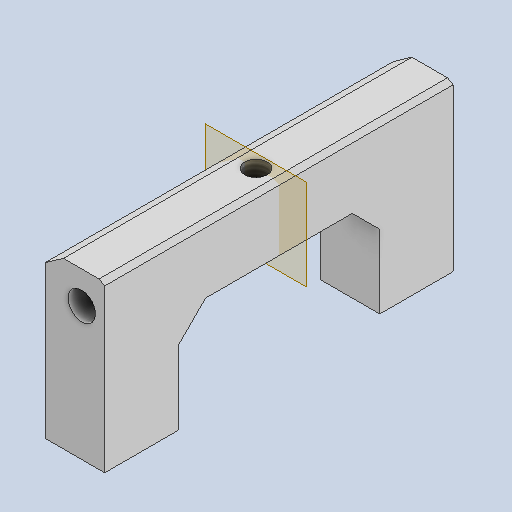
# Autodesk Inventor part: daVincihead_Sled_ToolAufnahmeBuegel_38mm
Saved by Autodesk Inventor 2024 (Build 280153000, 153)
## iProperties
Created: 2022-08-16
Part Number: daVincihead_Sled_ToolAufnahmeBuegel_38mm
Material: Generisch
Document SubType Name: Modeling
Designer: alexw
Density: 1 g/cm^3
Appearance: Vorgabe
Mass: 2.50955 g
Surface Area: 21.9008 cm^2
Volume: 2.50955 cm^3
Author: alexw
Autodesk Inventor part; units mm, degrees
ref_plane "YZ Plane" through (0, 0, 0) normal (1, 0, 0) x (0, 1, 0)
ref_plane "XZ Plane" through (0, 0, 0) normal (0, 1, 0) x (-1, 0, 0)
ref_plane "XY Plane" through (0, 0, 0) normal (0, 0, 1) x (1, 0, 0)
sketch "Skizze1" plane through (0, 0, 0) normal (0, 0, 1) x (1, 0, 0)
  line L0 (-4, 3.5) -> (4, 3.5)
  line L1 (4, 3.5) -> (4, -3.5)
  line L2 (4, -3.5) -> (-4, -3.5)
  line L3 (-4, -3.5) -> (-4, 3.5)
  line L4 (-4, 3.5) -> (4, -3.5) construction
  line L5 (4, 3.5) -> (-4, -3.5) construction
  line L6 (-4, 2.0996) -> (-2, 3.5)
  line L7 (1.8856, 3.5) -> (4, 2.2792)
  circle A0 centre (0, 0) radius 1.5
  line L8 (2.5, -3.5) -> (2.5, 3.5)
  point P0 (2.5, 3.1453)
  dimension "d0" = 35
  dimension "d1" = 2
  dimension "d2" = 7
  dimension "d3" = 8
  dimension "d4" = 30
  dimension "d5" = 3
  dimension "d31" = 2.5
  constraints: 18 end point, 6 point on line, 2 midpoint, 2 parallel, 2 perpendicular, 1 centre point, 1 coincident, 1 equal length, 1 horizontal
  measures "d0" angle of L0 L6
  measures "d1" horizontal distance of L6.end L6.start
  measures "d2" distance between parallel lines of L0 L2
  measures "d3" distance between parallel lines of L1 L3
  measures "d4" angle of L0 L7
  measures "d5" diameter of A0
  measures "d31" distance from line of L8 point (0, 0)
extrude "Extrusion1" add sketch "Skizze1" along normal blind 38 contours L0 L7 L8 L2 L3 L6 | L7 L1 L2 L8
ref_plane "Arbeitsebene1" through (0, 0, 19) normal (0, 0, 1) x (1, 0, 0)
sketch "Skizze2" plane through (-4, -3.5, 0) normal (0, -1, 0) x (1, 0, 0)
  line L0 (0, 0) -> (8, 0)
  line L1 (8, 0) -> (8, 8)
  line L2 (8, 8) -> (0, 8)
  line L3 (0, 8) -> (0, 0)
  line L4 (0, 0) -> (8, 8) construction
  line L5 (8, 0) -> (0, 8) construction
  line L6 (-1.6, 19) -> (9.6, 19) construction
  line L7 (4, 0) -> (4, 19) construction
  line L8 (0, 0) -> (0, 38) construction
  line L9 (8, 0) -> (8, 38) construction
  line L10 (0, 38) -> (8, 38)
  line L11 (8, 38) -> (8, 30)
  line L12 (8, 30) -> (0, 30)
  line L13 (0, 30) -> (0, 38)
  line L14 (0, 38) -> (8, 30) construction
  line L15 (8, 38) -> (0, 30) construction
  point P0 (4, 4)
  point P1 (4, 4)
  point P2 (4, 34)
  point P3 (4, 34)
  point P4 (4, 34)
  point P5 (4, 4)
  point P6 (4, 4)
  dimension "d8" = 8
  dimension "d9" = 8
  dimension "d29" = 30
  constraints: 26 end point, 7 midpoint, 6 symmetric about line, 2 coincident, 2 parallel, 2 perpendicular, 1 collinear, 1 horizontal, 1 point on line
  measures "d8" distance between parallel lines of L8 L9
  measures "d9" distance between parallel lines of L0 L2
  measures "d29" diameter of point (4, 4) L6
extrude "Extrusion2" add sketch "Skizze2" along normal blind 11
chamfer "Fase1" distance 3 angle 45 2 edges at (0, -3.5, 30) (0, -3.5, 8)
sketch "Skizze3" plane through (-4, -14.5, 0) normal (0, -1, 0) x (1, 0, 0)
  point P0 (4, 0)
  point P1 (4, 34)
  point P2 (4, 4)
hole "Bohrung1" at (0, -14.5, 34) at (0, -14.5, 4) direction (0, 1, 0) diameter 2.459 depth 8.8 tip angle 118 thread size "M3x0.5" class "6H" standard "ISO Metric profile"
sketch "Skizze4" plane through (-2, 3.5, 0) normal (0, 1, 0) x (1, 0, 0)
  line L0 (7.6, -19) -> (-3.6, -19) construction
  line L1 (2, -19) -> (2, 0) construction
  constraints: 2 end point, 1 midpoint, 1 vertical
hole "Bohrung2" at (0, 3.5, 19) direction (0, -1, 0) diameter 2.459 end up to surface thread size "M3x0.5" class "6H" standard "ISO Metric profile"
extrude "Extrusion3" cut sketch "Skizze1" along normal through all contours L7 L1 L2 L8
delete faces "Fläche löschen1" heal yes whole lump no faces at (3, -3.5, 30.6667) (3.5, -3.5, 7.3333)
equation "\"d9\" = d8"
